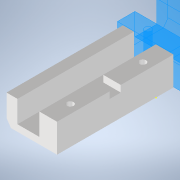
# Autodesk Inventor part: PiezaAtras
Saved by Autodesk Inventor 2021 (Build 250183000, 183)
## iProperties
Created: 2021-10-29
Part Number: PiezaAtras
Material: Genérico
Document SubType Name: Chapa
Designer: Juan Camilo
Density: 1 g/cm^3
Sheet Metal Rule: Por defecto_mm
Appearance: Valor por defecto
Author: Juan Camilo
Autodesk Inventor part; units mm, degrees
ref_plane "YZ Plane" through (0, 0, 0) normal (1, 0, 0) x (0, 1, 0)
ref_plane "XZ Plane" through (0, 0, 0) normal (0, 1, 0) x (-1, 0, 0)
ref_plane "XY Plane" through (0, 0, 0) normal (0, 0, 1) x (1, 0, 0)
sketch "Boceto1" plane through (0, 0, 0) normal (0, 1, 0) x (-1, 0, 0)
  line L0 (9.0356, 45.002) -> (-13.9644, 45.002)
  line L1 (-13.9644, 45.002) -> (-13.9644, -7.998)
  line L2 (-13.9644, -7.998) -> (9.0356, -7.998)
  line L3 (9.0356, -7.998) -> (9.0356, 45.002)
  point P0 (0, 0)
  dimension "d0" = 23
  dimension "d1" = 53
  constraints: 8 end point, 2 parallel, 1 horizontal, 1 perpendicular
  measures "d0" distance of L1.end L2.end
  measures "d1" distance of L0.end L1.end
extrude "Extrusión1" add sketch "Boceto1" along normal blind 3
sketch "Boceto2" plane through (0, 3, 0) normal (0, 1, 0) x (1, 0, 0)
  line L0 (-9.0356, -45.002) -> (13.9644, -45.002) projected
  line L1 (13.9644, -45.002) -> (13.9644, 7.998) projected
  line L2 (5.9644, -45.002) -> (13.9644, -45.002)
  line L3 (13.9644, -45.002) -> (13.9644, 7.998)
  line L4 (13.9644, 7.998) -> (5.9644, 7.998)
  line L5 (5.9644, 7.998) -> (5.9644, -45.002)
  point P0 (0, 0)
  dimension "d4" = 8
  constraints: 8 end point, 2 parallel, 1 horizontal, 1 perpendicular, 1 point on line
  measures "d4" distance of L1.end L4.end
extrude "Extrusión2" add sketch "Boceto2" along normal blind 10
sketch "Boceto3" plane through (0, 13, 0) normal (0, 1, 0) x (1, 0, 0)
  line L0 (5.9644, 7.998) -> (5.9644, -45.002) projected
  line L1 (5.9644, -21.002) -> (13.9831, -21.002)
  line L2 (13.9831, -21.002) -> (13.9831, -16.002)
  line L3 (13.9831, -16.002) -> (5.9644, -16.002)
  line L4 (5.9644, -16.002) -> (5.9644, -21.002)
  line L5 (13.9644, 7.998) -> (5.9644, 7.998) projected
  line L6 (5.9644, -45.002) -> (13.9644, -45.002) projected
  point P0 (0, 0)
  dimension "d7" = 24
  dimension "d8" = 5
  dimension "d9" = 24
  constraints: 8 end point, 2 parallel, 1 horizontal, 1 perpendicular, 1 point on line
  measures "d7" distance between parallel lines of L5 L3
  measures "d8" distance between parallel lines of L3 L1
  measures "d9" distance between parallel lines of L6 L1
extrude "Extrusión3" cut sketch "Boceto3" against normal blind 3
sketch "Boceto4" plane through (0, 13, 0) normal (0, 1, 0) x (1, 0, 0)
  circle A0 centre (9.9644, -2.002) radius 1.5
  line L0 (13.9644, 7.998) -> (5.9644, 7.998) projected
  line L1 (13.9644, -16.002) -> (13.9644, 7.998) projected
  line L2 (13.9644, -45.002) -> (13.9644, 7.998) projected
  line L3 (13.9644, -18.502) -> (5.9644, -18.502)
  circle A1 centre (9.9644, -35.002) radius 1.5
  point P0 (0, 0)
  dimension "d12" = 3
  dimension "d13" = 10
  dimension "d14" = 4
  constraints: 2 centre point, 2 end point, 1 horizontal, 1 midpoint, 1 symmetric about line, 1 other
  measures "d12" diameter of A0
  measures "d13" distance from line of L0 A0.centre
  measures "d14" distance from line of L1 A0.centre
extrude "Extrusión4" cut sketch "Boceto4" against normal blind 14.75
sketch "Boceto5" plane through (0, 3, 0) normal (0, 1, 0) x (1, 0, 0)
  line L0 (-9.0356, -45.002) -> (-4.0356, -45.002)
  line L1 (-4.0356, -45.002) -> (-4.0356, 7.998)
  line L2 (-4.0356, 7.998) -> (-9.0356, 7.998)
  line L3 (-9.0356, 7.998) -> (-9.0356, -45.002)
  point P0 (0, 0)
  dimension "d17" = 5
  constraints: 8 end point, 2 parallel, 1 horizontal, 1 perpendicular
  measures "d17" distance of L0.start L0.end
extrude "Extrusión5" add sketch "Boceto5" along normal blind 10
sketch "Boceto7" plane through (13.9644, 0, -7.998) normal (0, 0, -1) x (-1, 0, 0)
  line L0 (23, 0) -> (21, 0)
  line L1 (23, 0) -> (0, 0) projected
  line L2 (23, 0) -> (23, 3)
  line L3 (21, 0) -> (23, 3)
  point P0 (13.9644, 0)
  dimension "d24" = 2
  dimension "d25" = 3
  constraints: 6 end point, 1 point on line
  measures "d24" distance of L0.start L0.end
  measures "d25" distance of L0.start L2.end
extrude "Extrusión7" cut sketch "Boceto7" against normal blind 55.5
sketch "Boceto8" plane through (13.9644, 0, 45.002) normal (1, 0, 0) x (0, 0, -1)
  point P0 (45.002, 0)
equation "\"Radio_pliegue\" = Grosor"
equation "\"Anchura_desahogo_plegado\" = Grosor"
equation "\"Profundidad_desahogo_plegado\" = 0.5 * Grosor"
equation "\"Tamaño_destalonado\" = 4 * Grosor"
equation "\"Remanente_mínimo\" = 2 * Grosor"
equation "\"Radiodetransición\" = Radio_pliegue"
equation "\"Tamaño_de_radio_de_Jacobi\" = Radio_pliegue"
equation "\"TamañoSeparación\" = Grosor"
equation "\"Grosor\" = 0.5"
